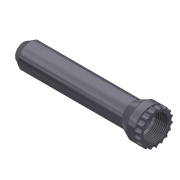
# Autodesk Inventor part: Head03
Saved by Autodesk Inventor 2019 (Build 230136000, 136)
## iProperties
Company: RIVETEC s.r.o.
Category: Naradi
Created: 2015-07-23
Part Number: Head03
Material: ETG 100
Description: přední hubice
Vendor: RIVETEC s.r.o.
Document SubType Name: Modeling
Designer: Solfronk
Stock Number: 10-1861
Mass: 90.1031 g
Surface Area: 117.934 cm^2
Volume: 11.4927 cm^3
Density: 7.84 g/cm^3
Appearance: Kov-Ocel (lesklá) mat
Hrubá hmotnost: 0
VV: 00
NázevAnglicky: PART
Datum uložení: 2009-01-26
Čas uložení: 09:36
Jméno souboru: RIVETEC
LastSaveDate: 2016-11-23
Mass: 0.1
FileName: P00000138
Plocha: =<SurfaceArea> /cm2
Objem: =<Volume> /cm3
Tolerance: ISO 2768-mK
Povrch_u: ČERNIT
Author: Solfronk
Revision Number: -
Last Saved By: navara
Autodesk Inventor part; units mm, degrees
ref_plane "YZ Plane" through (0, 0, 0) normal (1, 0, 0) x (0, 1, 0)
ref_plane "XZ Plane" through (0, 0, 0) normal (0, 1, 0) x (-1, 0, 0)
ref_plane "XY Plane" through (0, 0, 0) normal (0, 0, 1) x (1, 0, 0)
sketch "Náčrt1" plane through (0, 0, 0) normal (0, 0, 1) x (1, 0, 0)
  line L0 (0, 0) -> (-120, 0)
  line L1 (-120, 0) -> (-120, 11)
  line L2 (-120, 11) -> (-20.578, 11)
  line L3 (-20.578, 11) -> (-12, 15)
  line L4 (-12, 15) -> (0, 15)
  line L5 (0, 15) -> (0, 0)
  dimension "d2" = 22
  dimension "d3" = 30
  dimension "d4" = 12
  dimension "d5" = 25
  dimension "d6" = 120
  constraints: 12 end point, 3 perpendicular, 1 horizontal, 1 parallel
  measures "d2" diameter of L2 L0
  measures "d3" diameter of L4 L0
  measures "d4" distance from line of L3.end L5
  measures "d5" angle of L0 L3
  measures "d6" distance between parallel lines of L5 L1
revolve "Rotace1" add sketch "Náčrt1" angle 360 about axis through (0, 0, 0) along (-1, 0, 0)
hole "Díra1" at (0, 0, 0) direction (-1, 0, 0) diameter 22.38 depth 14 tip angle 118
hole "Díra2" at (0, 0, 0) direction (-1, 0, 0) diameter 19.2 depth 75 tip angle 118
hole "Díra3" at (-120, 0, 0) direction (1, 0, 0) diameter 8.92 depth 12 tip angle 118
chamfer "Zkosení1" distance 6 angle 30 1 edges at (-120, -11, 0) measured on face at (-53.7187, 10.8576, 1.7645)
sketch "Náčrt2" plane through (0, 0, 0) normal (1, 0, 0) x (0, 0, -1)
  circle A0 centre (16, 0) radius 2.6
  point P0 (0, 0)
  dimension "d40" = 16
  dimension "d41" = 5.2
  constraints: 1 centre point, 1 coincident
  measures "d40" distance of point (0, 0) point (16, 0)
  measures "d41" diameter of A0
extrude "Vysunutí1" cut sketch "Náčrt2" against normal blind 5
pattern_circular "Kruhové pole1" count 18 over 360 about axis through (-6, 0, 0) along (1, 0, 0) of "Vysunutí1"
chamfer "Zkosení2" distance 0.5 angle 45 1 edges at (0, 0, 11.19)
